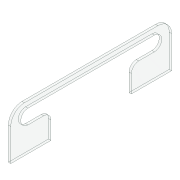
# Autodesk Inventor part: centralbar-210
Saved by Autodesk Inventor 2020 (Build 240168000, 168)
## iProperties
Created: 2021-06-22
Part Number: centralbar-210
Material: Generic
Document SubType Name: Modeling
Designer: Aidan Lee
Density: 1 g/cm^3
Appearance: Clear
Author: Aidan Lee
Autodesk Inventor part; units mm, degrees
ref_plane "YZ Plane" through (0, 0, 0) normal (1, 0, 0) x (0, 1, 0)
ref_plane "XZ Plane" through (0, 0, 0) normal (0, 1, 0) x (-1, 0, 0)
ref_plane "XY Plane" through (0, 0, 0) normal (0, 0, 1) x (1, 0, 0)
sketch "Sketch1" plane through (0, 0, 0) normal (1, 0, 0) x (0, 1, 0)
  line L0 (0, 0) -> (18, 0) construction
  line L1 (18, 0) -> (18, -390) construction
  line L2 (18, -390) -> (0, -390) construction
  line L3 (0, -390) -> (0, 0) construction
  line L4 (88, 0) -> (78, 0) construction
  line L5 (78, 0) -> (78, -210) construction
  line L6 (78, -210) -> (88, -210) construction
  line L7 (88, -210) -> (88, 0) construction
  line L8 (18, 0) -> (28, 0) construction
  line L9 (28, 0) -> (28, -210) construction
  line L10 (28, -210) -> (18, -210) construction
  line L11 (18, -210) -> (18, 0) construction
  circle A0 centre (53, -21.3494) radius 25 construction
  line L12 (28, 0) -> (13, 0) construction
  line L13 (13, 0) -> (13, -105) construction
  line L14 (13, -105) -> (28, -105) construction
  line L15 (28, 0) -> (35, 0) construction
  line L16 (35, 0) -> (35, -4) construction
  arc A1 (35, -4) -> (28, -11) centre (35, -11) ccw construction
  line L17 (28, -11) -> (28, -105) construction
  circle A2 centre (53, -21.3494) radius 4 construction
  circle A3 centre (53, -188.6506) radius 25 construction
  circle A4 centre (53, -188.6506) radius 4 construction
  line L18 (57, -21.3494) -> (57, 53.377) construction
  line L19 (44, -26.3494) -> (44, -46)
  arc A5 (35, -55) -> (44, -46) centre (35, -46) ccw
  line L20 (35, -55) -> (13, -55)
  line L21 (49, -21.3494) -> (49, -26.623) construction
  line L22 (53, -5) -> (13, -5)
  line L23 (13, -5) -> (13, -55)
  line L24 (70, -22) -> (70, -105)
  line L25 (62, -105) -> (62, -26.3494)
  arc A6 (44, -164) -> (35, -155) centre (35, -164) ccw
  line L26 (35, -155) -> (13, -155)
  line L27 (53, -205) -> (13, -205)
  line L28 (13, -205) -> (13, -155)
  arc A7 (62, -26.3494) -> (44, -26.3494) centre (53, -26.3494) ccw
  line L29 (53, -17.3494) -> (54.9283, -17.3494) construction
  line L30 (53, -17.3494) -> (54.5485, -17.3494) construction
  line L31 (44, -183.6506) -> (44, -164)
  line L32 (62, -105) -> (62, -183.6506)
  arc A8 (44, -183.6506) -> (62, -183.6506) centre (53, -183.6506) ccw
  line L33 (53, -21.3494) -> (53, -188.6506) construction
  line L34 (49, -21.3494) -> (49, -188.6506) construction
  line L35 (57, -188.6506) -> (57, -21.3494) construction
  arc A9 (57, -21.3494) -> (49, -21.3494) centre (53, -21.3494) ccw construction
  arc A10 (49, -188.6506) -> (57, -188.6506) centre (53, -188.6506) ccw construction
  arc A11 (70, -22) -> (53, -5) centre (53, -22) ccw
  line L36 (70, -188) -> (70, -105)
  arc A12 (53, -205) -> (70, -188) centre (53, -188) ccw
  point P0 (20.5, -105)
  point P1 (53, -105)
  dimension "d6" = 50
  dimension "d0" = 18
  dimension "d1" = 210
  dimension "d3" = 60
  dimension "d4" = 390
  dimension "d5" = 10
  dimension "d7" = 5
  dimension "d11" = 7
  dimension "d13" = 7
  dimension "d14" = 8
  dimension "d15" = 5
  dimension "d17" = 5
  dimension "d19" = 9
  dimension "d28" = 11
  dimension "d29" = 8
  dimension "d31" = 5
  dimension "d32" = 200
  dimension "d33" = 50
  dimension "d34" = 10
  dimension "d35" = 18
  constraints: 76 end point, 22 point on circle, 14 symmetric about line, 12 centre point, 10 tangent, 8 horizontal, 8 parallel, 8 vertical, 7 perpendicular, 5 horizontal alignment, 3 coincident, 3 collinear, 3 midpoint, 3 vertical alignment, 2 point on line, 1 concentric, 8 other
  measures "d0" distance of L0.start L0.end
  measures "d1" distance of L6.end L4.start
  measures "d3" distance between parallel lines of L5 L1
  measures "d4" distance of L2.end L0.start
  measures "d5" distance between parallel lines of L1 L9
  measures "d7" distance between parallel lines of L1 L13
  measures "d11" distance of L8.end L15.end
  measures "d13" radius of A1
  measures "d14" diameter of A2
  measures "d15" distance from line of L25.end L18
  measures "d17" distance between parallel lines of L19 L21
  measures "d19" radius of A5
  measures "d28" distance from line of L0 A1.centre
  measures "d29" distance between parallel lines of L25 L24
  measures "d31" distance between parallel lines of L8 L22
  measures "d32" distance between parallel lines of L27 L22
  measures "d33" distance of L22.end L20.end
  measures "d34" distance of L4.start L4.end
  measures "d35" distance between parallel lines of L36 L7
extrude "Extrusion2" add sketch "Sketch1" along normal blind 3
equation "\"d19\" = d18"
equation "\"d18\" = 9"
body "Solid2"
